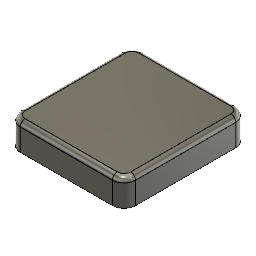
Top Housing (Autodesk Fusion 360 design; units mm, degrees)
Autodesk Fusion 360 part; units mm, degrees
ref_plane "WorkPlane1" through (0, -1, 0) normal (0, 1, 0) x (0, 0, 1)
sketch "Sketch2" plane through (0, -1, 0) normal (0, 1, 0) x (1, 0, 0)
  line L0 (-28, 3) -> (29.829, 3)
  line L1 (29.829, 3) -> (29.829, -59)
  line L2 (29.829, -59) -> (-28, -59)
  line L3 (-28, -59) -> (-28, 3)
  line L4 (28.829, -0.127) -> (28.829, -45.974)
  line L5 (0, -45.847) -> (0, -0.127)
  line L6 (-29, 4) -> (-29, -60)
  line L7 (-29, -60) -> (30.829, -60)
  line L8 (30.829, -60) -> (30.829, 4)
  line L9 (30.829, 4) -> (-29, 4)
  line L10 (0.127, 0) -> (28.702, 0)
  dimension "d2" = 1
  dimension "d3" = 28
  dimension "d4" = 62
  dimension "d7" = 1
  dimension "d8" = 1
  dimension "d9" = 3
  dimension "d10" = 1
  dimension "d11" = 1
  measures "d2" distance of L1 L4
  measures "d3" distance of L3 L5
  measures "d4" distance of origin
  measures "d7" distance of L0 L9
  measures "d8" distance of L1 L8
  measures "d9" distance of L0 L10
  measures "d10" distance of L2 L7
  measures "d11" distance of L3 L6
extrude "Extrude2" add sketch "Sketch2" against normal blind 1.5 contours L0 L1 L2 L3 | L6 L7 L8 L9
sketch "Sketch3" plane through (0, -1, 0) normal (0, 1, 0) x (1, 0, 0)
  circle A0 centre (25.829, -55) radius 2.5
  line L0 (29.829, 3) -> (29.829, -59)
  line L1 (29.829, -59) -> (-28, -59)
  line L2 (-28, -59) -> (-28, 3)
  line L3 (-28, -28) -> (29.829, -28)
  circle A1 centre (25.829, -1) radius 2.5
  line L4 (-28, 3) -> (29.829, 3)
  line L5 (0.9145, 3) -> (0.9145, -59)
  circle A2 centre (-24, -1) radius 2.5
  circle A3 centre (-24, -55) radius 2.5
  dimension "d14" = 5
  dimension "d15" = 4
  dimension "d16" = 4
  measures "d14" diameter of A0
  measures "d15" distance of origin L0
extrude "Extrude3" add sketch "Sketch2" sketch "Sketch3" along normal blind 12.5 of sketch 2 contours A0 | A1 | A2 | A3
fillet "Fillet1" radius 5 1 edges at (-28, 5.25, -3)
fillet "Fillet2" radius 6 1 edges at (-29, 4.5, -4)
fillet "Fillet3" radius 5.5 1 edges at (-28, 5.25, 59)
fillet "Fillet4" radius 6 1 edges at (-29, 4.5, 60)
fillet "Fillet5" radius 5 1 edges at (29.829, 5.25, -3)
fillet "Fillet6" radius 6 1 edges at (30.829, 4.5, -4)
fillet "Fillet7" radius 5 1 edges at (29.829, 5.25, 59)
fillet "Fillet8" radius 6 1 edges at (30.829, 4.5, 60)
fillet "Fillet9" radius 2.5 8 edges at (-27.2426, -2.5, 58.2426) (-29, -2.5, 28) (-27.2426, -2.5, -2.2426) (0.9145, -2.5, -4) (29.0716, -2.5, -2.2426) (30.829, -2.5, 28) (29.0716, -2.5, 58.2426) (0.9145, -2.5, 60) 1 faces at (10.886, -2.5, 36.6667)
ref_plane "WorkPlane2" through (0, 12.2, 0) normal (0, 1, 0) x (0, 0, 1)
move_body "Move3" bodies 1 to x (-1, 0, 0) y (0, -1, 0) z (0, 0, 1) at (0, 0, 0)
move_body "Move4" bodies 1 to x (1, 0, 0) y (0, 1, 0) z (0, 0, 1) at (0, 12.2, 0)
sketch "Sketch8" plane through (0, 0.7, 0) normal (0, -1, 0) x (1, 0, 0)
  circle A0 centre (-25.829, 1) radius 2.5
  circle A1 centre (-25.829, 1) radius 2.5
  circle A2 centre (24, 1) radius 2.5
  circle A3 centre (-25.829, 55) radius 2.5
  circle A4 centre (24, 55) radius 2.5
hole "Hole1" at (-25.829, 0.7, 1) at (24, 0.7, 1) at (-25.829, 0.7, 55) at (24, 0.7, 55) direction (0, 1, 0) diameter 2.93 depth 10 tip angle 180
thread "Thread1" "ISO Metric profile 3.5 M3.5x0.6 6H"
